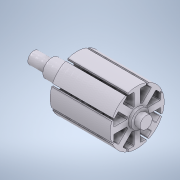
# Autodesk Inventor part: Motor_rotor
Saved by Autodesk Inventor 2021 (Build 250183000, 183)
## iProperties
Created: 2021-07-09
Part Number: Motor_rotor
Material: Aluminum 6061, Welded
Document SubType Name: Modeling
Designer: MOGIRE
Density: 2.7 g/cm^3
Appearance: Weld - Aluminum
Author: MOGIRE
Autodesk Inventor part; units mm, degrees
ref_plane "YZ Plane" through (0, 0, 0) normal (1, 0, 0) x (0, 1, 0)
ref_plane "XZ Plane" through (0, 0, 0) normal (0, 1, 0) x (-1, 0, 0)
ref_plane "XY Plane" through (0, 0, 0) normal (0, 0, 1) x (1, 0, 0)
sketch "Sketch1" plane through (0, 0, 0) normal (1, 0, 0) x (0, 1, 0)
  circle A0 centre (0, 0) radius 50
  dimension "d0" = 100
  constraints: 1 centre point, 1 coincident
  measures "d0" diameter of A0
extrude "Extrusion1" add sketch "Sketch1" along normal blind 150
sketch "Sketch2" plane through (150, 0, 0) normal (1, 0, 0) x (0, 0, -1)
  circle A0 centre (0, 0) radius 75
  dimension "d3" = 150
  constraints: 1 centre point, 1 coincident
  measures "d3" diameter of A0
extrude "Extrusion2" add sketch "Sketch2" along normal blind 210
sketch "Sketch3" plane through (360, 0, 0) normal (1, 0, 0) x (0, 0, -1)
  arc A0 (76.2887, 211.672) -> (-75.5618, 211.9326) centre (0, 0) ccw construction
  line L0 (0, 0) -> (0, 225) construction
  line L1 (0, 225) -> (26.2887, 225)
  line L2 (0, 225) -> (-26.2887, 225)
  line L3 (76.2887, 211.672) -> (76.2887, 200.0277)
  line L4 (71.2887, 195.0277) -> (31.2887, 195.0277)
  line L5 (0, 225) -> (-26.2887, 225)
  line L6 (-71.199, 195.0277) -> (-31.2887, 195.0277)
  arc A1 (-76.199, 197.1136) -> (-74.2008, 195.0277) centre (-74.2008, 197.0277) ccw
  circle A2 centre (0, 0) radius 225
  line L7 (-26.2887, 86.075) -> (-26.2887, 190.0277)
  line L8 (-75, 212.132) -> (-75, 225)
  line L9 (26.2887, 86.075) -> (26.2887, 190.0277)
  line L10 (75, 212.132) -> (75, 225)
  arc A3 (-76.199, 197.1136) -> (-74.2008, 195.0277) centre (-74.2008, 197.0277) ccw
  line L11 (-76.199, 200.0277) -> (-76.199, 211.7043)
  arc A4 (-26.2887, 193.0277) -> (-28.2887, 195.0277) centre (-28.2887, 193.0277) ccw
  arc A5 (28.2887, 195.0277) -> (26.2887, 193.0277) centre (28.2887, 193.0277) ccw
  arc A6 (-76.199, 197.0277) -> (-74.199, 195.0277) centre (-74.199, 197.0277) ccw
  arc A7 (-26.2887, 190.0277) -> (-31.2887, 195.0277) centre (-31.2887, 190.0277) ccw
  arc A8 (31.2887, 195.0277) -> (26.2887, 190.0277) centre (31.2887, 190.0277) ccw
  arc A9 (71.2887, 195.0277) -> (76.2887, 200.0277) centre (71.2887, 200.0277) ccw
  arc A10 (-76.199, 200.0277) -> (-71.199, 195.0277) centre (-71.199, 200.0277) ccw
  line L12 (0, 0) -> (159.099, 159.099) construction
  line L13 (0, 0) -> (225, 0) construction
  arc A11 (-75.5618, -211.9326) -> (76.2887, -211.672) centre (0, 0) ccw construction
  line L14 (76.2887, -211.672) -> (76.2887, -200.0277)
  line L15 (71.2887, -195.0277) -> (31.2887, -195.0277)
  line L16 (-71.199, -195.0277) -> (-31.2887, -195.0277)
  line L17 (-26.2887, -86.075) -> (-26.2887, -190.0277)
  line L18 (26.2887, -86.075) -> (26.2887, -190.0277)
  line L19 (-76.199, -200.0277) -> (-76.199, -211.7043)
  arc A12 (-31.2887, -195.0277) -> (-26.2887, -190.0277) centre (-31.2887, -190.0277) ccw
  arc A13 (26.2887, -190.0277) -> (31.2887, -195.0277) centre (31.2887, -190.0277) ccw
  arc A14 (76.2887, -200.0277) -> (71.2887, -195.0277) centre (71.2887, -200.0277) ccw
  line L20 (211.672, 76.2887) -> (200.0277, 76.2887)
  line L21 (195.0277, 71.2887) -> (195.0277, 31.2887)
  line L22 (195.0277, -71.199) -> (195.0277, -31.2887)
  line L23 (86.075, -26.2887) -> (190.0277, -26.2887)
  line L24 (86.075, 26.2887) -> (190.0277, 26.2887)
  line L25 (200.0277, -76.199) -> (211.7043, -76.199)
  arc A15 (195.0277, -31.2887) -> (190.0277, -26.2887) centre (190.0277, -31.2887) ccw
  arc A16 (200.0277, 76.2887) -> (195.0277, 71.2887) centre (200.0277, 71.2887) ccw
  arc A17 (195.0277, -71.199) -> (200.0277, -76.199) centre (200.0277, -71.199) ccw
  arc A18 (195.0277, -31.2887) -> (190.0277, -26.2887) centre (190.0277, -31.2887) ccw
  arc A19 (190.0277, 26.2887) -> (195.0277, 31.2887) centre (190.0277, 31.2887) ccw
  line L26 (-86.075, -26.2887) -> (-190.0277, -26.2887)
  line L27 (-86.075, 26.2887) -> (-190.0277, 26.2887)
  line L28 (-195.0277, 71.2887) -> (-195.0277, 31.2887)
  arc A20 (-195.0277, 71.2887) -> (-200.0277, 76.2887) centre (-200.0277, 71.2887) ccw
  line L29 (-211.672, 76.2887) -> (-200.0277, 76.2887)
  line L30 (-195.0277, -71.199) -> (-195.0277, -31.2887)
  arc A21 (-190.0277, -26.2887) -> (-195.0277, -31.2887) centre (-190.0277, -31.2887) ccw
  line L31 (-200.0277, -76.199) -> (-211.7043, -76.199)
  arc A22 (-200.0277, -76.199) -> (-195.0277, -71.199) centre (-200.0277, -71.199) ccw
  arc A23 (-195.0277, 31.2887) -> (-190.0277, 26.2887) centre (-190.0277, 31.2887) ccw
  line L32 (0, 0) -> (207.8729, 86.1038) construction
  line L33 (0, 0) -> (225, 0) construction
  line L34 (42.2753, 79.4531) -> (115.781, 152.9588)
  line L35 (79.4531, 42.2753) -> (152.9588, 115.781)
  line L36 (188.3141, 87.4967) -> (160.0298, 115.781)
  arc A24 (188.3141, 87.4967) -> (195.3852, 87.4967) centre (191.8496, 91.0322) ccw
  line L37 (203.6189, 95.7305) -> (195.3852, 87.4967)
  line L38 (87.5601, 188.2507) -> (115.781, 160.0298)
  arc A25 (115.781, 152.9588) -> (115.781, 160.0298) centre (112.2454, 156.4943) ccw
  line L39 (87.5601, 195.3217) -> (95.8167, 203.5784)
  arc A26 (87.5601, 195.3217) -> (87.5601, 188.2507) centre (91.0957, 191.7862) ccw
  arc A27 (160.0298, 115.781) -> (152.9588, 115.781) centre (156.4943, 112.2454) ccw
  line L40 (86.075, 26.2887) -> (190.0277, 26.2887)
  line L41 (86.075, -26.2887) -> (190.0277, -26.2887)
  line L42 (195.0277, -71.2887) -> (195.0277, -31.2887)
  arc A28 (195.0277, -71.2887) -> (200.0277, -76.2887) centre (200.0277, -71.2887) ccw
  line L43 (211.672, -76.2887) -> (200.0277, -76.2887)
  line L44 (195.0277, 71.199) -> (195.0277, 31.2887)
  arc A29 (190.0277, 26.2887) -> (195.0277, 31.2887) centre (190.0277, 31.2887) ccw
  line L45 (200.0277, 76.199) -> (211.7043, 76.199)
  arc A30 (200.0277, 76.199) -> (195.0277, 71.199) centre (200.0277, 71.199) ccw
  arc A31 (195.0277, -31.2887) -> (190.0277, -26.2887) centre (190.0277, -31.2887) ccw
  line L46 (79.4531, -42.2753) -> (152.9588, -115.781)
  line L47 (42.2753, -79.4531) -> (115.781, -152.9588)
  line L48 (87.5601, -188.2507) -> (115.781, -160.0298)
  arc A32 (87.5601, -188.2507) -> (87.5601, -195.3217) centre (91.0957, -191.7862) ccw
  line L49 (87.5601, -195.3217) -> (95.8167, -203.5784)
  line L50 (188.3141, -87.4967) -> (160.0298, -115.781)
  arc A33 (152.9588, -115.781) -> (160.0298, -115.781) centre (156.4943, -112.2454) ccw
  line L51 (203.6189, -95.7305) -> (195.3852, -87.4967)
  arc A34 (195.3852, -87.4967) -> (188.3141, -87.4967) centre (191.8496, -91.0322) ccw
  arc A35 (115.781, -160.0298) -> (115.781, -152.9588) centre (112.2454, -156.4943) ccw
  line L52 (-42.2753, -79.4531) -> (-115.781, -152.9588)
  line L53 (-79.4531, -42.2753) -> (-152.9588, -115.781)
  arc A36 (-160.0298, -115.781) -> (-152.9588, -115.781) centre (-156.4943, -112.2454) ccw
  line L54 (-188.3141, -87.4967) -> (-160.0298, -115.781)
  line L55 (-203.6189, -95.7305) -> (-195.3852, -87.4967)
  arc A37 (-188.3141, -87.4967) -> (-195.3852, -87.4967) centre (-191.8496, -91.0322) ccw
  arc A38 (-115.781, -152.9588) -> (-115.781, -160.0298) centre (-112.2454, -156.4943) ccw
  line L56 (-87.5601, -188.2507) -> (-115.781, -160.0298)
  line L57 (-87.5601, -195.3217) -> (-95.8167, -203.5784)
  arc A39 (-87.5601, -195.3217) -> (-87.5601, -188.2507) centre (-91.0957, -191.7862) ccw
  line L58 (-42.2753, 79.4531) -> (-115.781, 152.9588)
  line L59 (-79.4531, 42.2753) -> (-152.9588, 115.781)
  line L60 (-188.3141, 87.4967) -> (-160.0298, 115.781)
  arc A40 (-152.9588, 115.781) -> (-160.0298, 115.781) centre (-156.4943, 112.2454) ccw
  line L61 (-203.6189, 95.7305) -> (-195.3852, 87.4967)
  arc A41 (-195.3852, 87.4967) -> (-188.3141, 87.4967) centre (-191.8496, 91.0322) ccw
  line L62 (-87.5601, 188.2507) -> (-115.781, 160.0298)
  arc A42 (-115.781, 160.0298) -> (-115.781, 152.9588) centre (-112.2454, 156.4943) ccw
  line L63 (-87.5601, 195.3217) -> (-95.8167, 203.5784)
  arc A43 (-87.5601, 188.2507) -> (-87.5601, 195.3217) centre (-91.0957, 191.7862) ccw
  arc A44 (-79.4531, 42.2753) -> (-86.075, 26.2887) centre (0, 0) ccw
  arc A45 (-86.075, -26.2887) -> (-79.4531, -42.2753) centre (0, 0) ccw
  arc A46 (-42.2753, -79.4531) -> (-26.2887, -86.075) centre (0, 0) ccw
  arc A47 (26.2887, -86.075) -> (42.2753, -79.4531) centre (0, 0) ccw
  arc A48 (79.4531, -42.2753) -> (86.075, -26.2887) centre (0, 0) ccw
  arc A49 (90, 0) -> (79.4531, 42.2753) centre (0, 0) ccw
  arc A50 (42.2753, 79.4531) -> (26.2887, 86.075) centre (0, 0) ccw
  arc A51 (-26.2887, 86.075) -> (-42.2753, 79.4531) centre (0, 0) ccw
  line L64 (-76.199, -200.0277) -> (-76.199, -200.0277)
  line L65 (-71.199, -195.0277) -> (-71.199, -195.0277)
  arc A52 (-71.199, -195.0277) -> (-76.199, -200.0277) centre (-71.199, -200.0277) ccw
  point P0 (76.2887, 195.0277)
  point P1 (26.2887, 195.0277)
  point P2 (-76.2887, 195.0277)
  point P3 (-26.2887, 195.0277)
  dimension "d6" = 450
  dimension "d10" = 75
  dimension "d11" = 75
  dimension "d12" = 30
  dimension "d13" = 2
  dimension "d14" = 2
  dimension "d15" = 2
  dimension "d16" = 2
  dimension "d17" = 5
  dimension "d18" = 225
  dimension "d19" = 45
  dimension "d20" = 225
  dimension "d21" = 22.5
  dimension "d24" = 5
  constraints: 132 end point, 131 symmetric about line, 110 point on circle, 53 centre point, 19 point on line, 19 tangent, 5 equal radius, 5 horizontal, 5 parallel, 4 vertical, 3 coincident, 2 equal length, 2 perpendicular, 33 other
  measures "d6" diameter of A0
  measures "d10" horizontal distance of point (0, 0) L10.end
  measures "d11" distance of L0.end L8.end
  measures "d12" distance of L10.end point (76.289, 195.028)
  measures "d13" radius of A1
  measures "d14" radius of A3
  measures "d15" radius of A4
  measures "d16" radius of A6
  measures "d17" radius of A7
  measures "d18" distance of L12.start L12.end
  measures "d19" angle of L13 L12
  measures "d20" distance of L12.start L32.end
  measures "d21" angle of L33 L32
  measures "d24" radius of A52
extrude "Extrusion3" add sketch "Sketch3" along normal blind 500 contours L3 A9 L4 A8 L9 A50 L34 A25 L38 A26 L39 A2 L37 A24 L36 A27 L35 A49 L24 A19 L21 A30 L45 L25 A17 L22 A15 L23 A48 L46 A33 L50 A34 L51 L49 A32 L48 A35 L47 A47 L18 A13 L15 A14 L14 L19 A52 L16 A12 L17 A46 L52 A38 L56 A39 L57 L55 A37 L54 A36 L53 A45 L26 A21 L30 A22 L31 L29 A20 L28 A23 L27 A44 L59 A40 L60 A41 L61 L63 A43 L62 A42 L58 A51 L7 A7 L6 A10 L11
sketch "Sketch6" plane through (860, 0, 0) normal (1, 0, 0) x (0, 0, -1)
  circle A0 centre (0, 0) radius 75
  dimension "d25" = 150
  constraints: 1 centre point, 1 coincident
  measures "d25" diameter of A0
extrude "Extrusion4" add sketch "Sketch6" along normal blind 25
sketch "Sketch7" plane through (885, 0, 0) normal (1, 0, 0) x (0, 0, -1)
  circle A0 centre (0, 0) radius 50
  dimension "d28" = 100
  constraints: 1 centre point, 1 coincident
  measures "d28" diameter of A0
extrude "Extrusion5" add sketch "Sketch7" along normal blind 50
equation "\"d11\" = d10"
body "Solid1"
